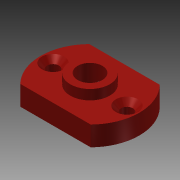
# Autodesk Inventor part: 13_1087_028
Saved by Autodesk Inventor 2014 (Build 180170000, 170)
## iProperties
Created: 2013-09-17
Part Number: 13_1087_028
Material: Allgemein
Document SubType Name: Modeling
Designer: vogel
Density: 1 g/cm^3
Appearance: Orangerot
Author: vogel
Autodesk Inventor part; units mm, degrees
note: some values were not read from the file. Chosen so that the rebuilt part matches the saved one: direction of "Bohrung1".
ref_plane "YZ Plane" through (0, 0, 0) normal (1, 0, 0) x (0, 1, 0)
ref_plane "XZ Plane" through (0, 0, 0) normal (0, 1, 0) x (-1, 0, 0)
ref_plane "XY Plane" through (0, 0, 0) normal (0, 0, 1) x (1, 0, 0)
sketch "Skizze1" plane through (0, 0, 0) normal (0, 0, 1) x (1, 0, 0)
  line L0 (-14, 0) -> (14, 0) projected
  line L1 (0, -14) -> (0, 14) projected
  circle A0 centre (0, 0) radius 10
  circle A1 centre (0, 0) radius 2.5
  dimension "d0" = 5
  dimension "d1" = 20
  constraints: 2 centre point, 2 coincident
  measures "d0" diameter of A1
  measures "d1" diameter of A0
extrude "Extrusion1" add sketch "Skizze1" along normal blind 5 contours A1 L1 A0 L0 | L0 A0 L1 A1 | A1 L0 A0 L1 | L1 A0 L0 A1
sketch "Skizze2" plane through (0, 0, 5) normal (0, 0, 1) x (1, 0, 0)
  circle A0 centre (0, 0) radius 10 projected
  line L0 (-14, 0) -> (14, 0) projected
  line L1 (0, -14) -> (0, 14) projected
  line L2 (-7.1414, 7) -> (7.1414, 7)
  line L3 (7.1414, -7) -> (-7.1414, -7)
  dimension "d4" = 14
  constraints: 4 end point, 4 point on circle, 1 parallel, 1 perpendicular, 1 other
  measures "d4" distance between parallel lines of L3 L2
extrude "Extrusion2" cut sketch "Skizze2" against normal through all contours L2 L1 A0 | A0 L1 L3 | L1 L2 A0 | A0 L3 L1
sketch "Skizze3" plane through (-7.1414, 7, 5) normal (0, 1, 0) x (1, 0, 0)
  line L0 (0, 5) -> (14.2829, 5) projected
  line L1 (-6.8586, 5) -> (21.1414, 5) projected
  line L2 (7.1414, 6) -> (7.1414, -1) projected
  point P0 (7.1414, 5)
  point P1 (7.1414, 2.5)
  dimension "d7" = 2.5
  constraints: 1 midpoint
  measures "d7" distance from line of L0 point (7.141, 2.5)
hole "Bohrung1" at (0, 7, 2.5) direction (0, -1, 0) diameter 2.459 end up to surface thread size "M3x0.5" class "6H" standard "ISO Metric profile"
sketch "Skizze4" plane through (0, 0, 5) normal (0, 0, 1) x (1, 0, 0)
  circle A0 centre (0, 0) radius 2.5 projected
  line L0 (-14, 0) -> (14, 0) projected
  line L1 (0, -14) -> (0, 14) projected
  circle A1 centre (0, 0) radius 7.5
  point P0 (-7.5, 0)
  point P1 (7.5, 0)
  dimension "d15" = 15
  constraints: 2 point on circle, 2 point on line, 1 centre point, 1 coincident
  measures "d15" diameter of A1
hole "Bohrung2" at (-7.5, 0, 5) at (7.5, 0, 5) direction (0, 0, -1) diameter 2.4 end through all countersink diameter 4.5 countersink angle 90
sketch "Skizze5" plane through (0, 0, 5) normal (0, 0, 1) x (1, 0, 0)
  circle A0 centre (0, 0) radius 2.5 projected
  circle A1 centre (0, 0) radius 4
  dimension "d23" = 8
  constraints: 1 centre point, 1 coincident
  measures "d23" diameter of A1
extrude "Extrusion3" add sketch "Skizze5" along normal blind 2
